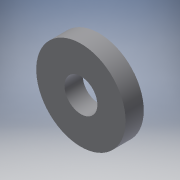
# Autodesk Inventor part: bearing
Saved by Autodesk Inventor 2019 (Build 230136000, 136)
## iProperties
Created: 2019-03-20
Part Number: bearing
Material: Generic
Document SubType Name: Modeling
Designer: s-4036947
Density: 1 g/cm^3
Appearance: Default
Author: s-4036947
Autodesk Inventor part; units mm, degrees
ref_plane "YZ Plane" through (0, 0, 0) normal (1, 0, 0) x (0, 1, 0)
ref_plane "XZ Plane" through (0, 0, 0) normal (0, 1, 0) x (-1, 0, 0)
ref_plane "XY Plane" through (0, 0, 0) normal (0, 0, 1) x (1, 0, 0)
sketch "Sketch1" plane through (0, 0, 0) normal (0, 0, 1) x (1, 0, 0)
  line L0 (0, 5.4993) -> (-4.7625, 2.7496) construction
  line L1 (-4.7625, 2.7496) -> (-4.7625, -2.7496) construction
  line L2 (-4.7625, -2.7496) -> (0, -5.4993) construction
  line L3 (0, -5.4993) -> (4.7625, -2.7496) construction
  line L4 (4.7625, -2.7496) -> (4.7625, 2.7496) construction
  line L5 (4.7625, 2.7496) -> (0, 5.4993) construction
  circle A0 centre (0, 0) radius 5.7493
  circle A1 centre (0, 0) radius 15.625
  circle A2 centre (-13.0717, -85.2567) radius 15.875 construction
  dimension "d0" = 5.4993
  dimension "d1" = 11.4985
  dimension "d2" = 31.75
  dimension "d3" = 31.25
  constraints: 2 centre point, 2 coincident
  measures "d0" distance of L2.end point (0, 0)
  measures "d1" diameter of A0
  measures "d2" diameter of A2
  measures "d3" diameter of A1
extrude "Extrusion1" add sketch "Sketch1" along normal blind 6.35
body "Solid1"
